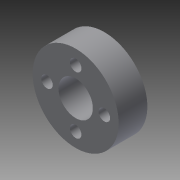
# Autodesk Inventor part: Bearing
Saved by Autodesk Inventor 2015 (Build 190159000, 159)
## iProperties
Created: 2016-04-14
Part Number: Bearing
Material: Generic
Document SubType Name: Modeling
Designer: Diogo Figueiredo
Density: 1 g/cm^3
Appearance: Default
Author: Diogo Figueiredo
Autodesk Inventor part; units mm, degrees
ref_plane "YZ Plane" through (0, 0, 0) normal (1, 0, 0) x (0, 1, 0)
ref_plane "XZ Plane" through (0, 0, 0) normal (0, 1, 0) x (-1, 0, 0)
ref_plane "XY Plane" through (0, 0, 0) normal (0, 0, 1) x (1, 0, 0)
sketch "Sketch1" plane through (0, 0, 0) normal (0, 1, 0) x (-1, 0, 0)
  circle A0 centre (0, 0) radius 15
  circle A1 centre (10, 0) radius 2
  circle A2 centre (0, -10) radius 2
  circle A3 centre (-10, 0) radius 2
  circle A4 centre (0, 10) radius 2
  circle A5 centre (0, 0) radius 6
  dimension "d0" = 30
  dimension "d2" = 4
  dimension "d3" = 4
  dimension "d4" = 4
  dimension "d5" = 4
  dimension "d6" = 12
  constraints: 6 centre point, 2 coincident
  measures "d0" diameter of A0
  measures "d2" diameter of A1
  measures "d3" diameter of A2
  measures "d4" diameter of A3
  measures "d5" diameter of A4
  measures "d6" diameter of A5
extrude "Extrusion1" add sketch "Sketch1" along normal blind 10
body "Solid1"
